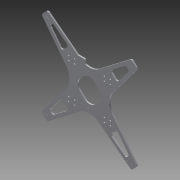
# Autodesk Inventor part: 6061 Bed holes no chamfer
Saved by Autodesk Inventor 2014 (Build 180170000, 170)
## iProperties
Created: 2016-05-10
Part Number: 6061 Bed holes no chamfer
Material: Aluminum 6061
Document SubType Name: Modeling
Designer: 101767
Density: 2.71 g/cm^3
Appearance: Aluminum - Flat
Mass: 1110.57 g
Surface Area: 1537.27 cm^2
Volume: 409.805 cm^3
Author: 101767
Autodesk Inventor part; units mm, degrees
ref_plane "YZ Plane" through (0, 0, 0) normal (1, 0, 0) x (0, 1, 0)
ref_plane "XZ Plane" through (0, 0, 0) normal (0, 1, 0) x (-1, 0, 0)
ref_plane "XY Plane" through (0, 0, 0) normal (0, 0, 1) x (1, 0, 0)
sketch "Plate" plane through (0, 0, 0) normal (0, 0, 1) x (1, 0, 0)
  line L0 (-200, -200) -> (200, -200) construction
  line L1 (200, -200) -> (200, 200) construction
  line L2 (200, 200) -> (-200, 200) construction
  line L3 (-200, 200) -> (-200, -200) construction
  line L4 (-200, -200) -> (200, 200) construction
  line L5 (200, -200) -> (-200, 200) construction
  line L6 (0, 0) -> (0, 420.657) construction
  line L7 (0, 0) -> (461.6465, 0) construction
  line L8 (0, 202) -> (202, 202) construction
  line L9 (202, 202) -> (202, 0) construction
  line L10 (74.8189, 0) -> (251.7605, 230.5948) construction
  line L11 (254.8388, 145.1612) -> (158.001, 241.999) construction
  line L12 (252.9755, 175.3088) -> (179.3809, 248.9034) construction
  line L13 (74.8189, 0) -> (228.2843, 200)
  line L14 (200, 200) -> (231.4665, 231.4665) construction
  line L15 (228.2843, 200) -> (214.1421, 214.1421)
  line L16 (200, 228.2843) -> (214.1421, 214.1421)
  line L17 (200, 228.2843) -> (0, 74.8189)
  line L18 (-74.8189, 0) -> (-228.2843, 200)
  line L19 (-228.2843, 200) -> (-214.1421, 214.1421)
  line L20 (-200, 228.2843) -> (-214.1421, 214.1421)
  line L21 (-200, 228.2843) -> (0, 74.8189)
  line L22 (74.8189, 0) -> (228.2843, -200)
  line L23 (228.2843, -200) -> (214.1421, -214.1421)
  line L24 (200, -228.2843) -> (214.1421, -214.1421)
  line L25 (200, -228.2843) -> (0, -74.8189)
  line L26 (-200, -228.2843) -> (0, -74.8189)
  line L27 (-200, -228.2843) -> (-214.1421, -214.1421)
  line L28 (-228.2843, -200) -> (-214.1421, -214.1421)
  line L29 (-74.8189, 0) -> (-228.2843, -200)
  dimension "d63" = 0
  dimension "d133" = 15
  dimension "d12" = 200
  dimension "d79" = 200
  dimension "d80" = 2
  dimension "d81" = 2
  dimension "d83" = 20
  dimension "d84" = 7.5
  dimension "d85" = 20
  dimension "d86" = 7.5
  constraints: 60 end point, 12 symmetric about line, 9 point on line, 5 parallel, 5 perpendicular, 2 midpoint, 1 horizontal
  measures "d12" distance between parallel lines of L7 L2
  measures "d79" distance from line of L1.end L6
  measures "d80" distance between parallel lines of L2 L8
  measures "d81" distance between parallel lines of L1 L9
  measures "d83" distance between parallel lines of L11 L12
  measures "d84" angle of L10 L4
  measures "d85" distance from line of L14 L13.end
  measures "d86" angle of L4 L17
extrude "Base" add sketch "Plate" along normal blind 6.35
sketch "Sketch3" plane through (0, 0, 0) normal (0, 0, 1) x (1, 0, 0)
  line L0 (-70.7107, 0) -> (0, 70.7107)
  line L1 (0, 70.7107) -> (70.7107, 0)
  line L2 (70.7107, 0) -> (0, -70.7107)
  line L3 (0, -70.7107) -> (-70.7107, 0)
  line L4 (-70.7107, 0) -> (70.7107, 0) construction
  line L5 (0, 70.7107) -> (0, -70.7107) construction
  point P0 (0, 0)
  dimension "d76" = 90
  dimension "d77" = 100
  constraints: 12 end point, 2 midpoint, 2 parallel, 1 perpendicular, 1 vertical
  measures "d76" angle of L4 L5
  measures "d77" distance of L0.end L1.end
extrude "Center hole" cut sketch "Sketch3" along normal through all
fillet "Fillet2" radius 75 4 edges at (0, 74.8189, 3.175) (-74.8189, 0, 3.175) (0, -74.8189, 3.175) (74.8189, 0, 3.175)
fillet "Fillet3" radius 35 4 edges at (-70.7107, 0, 3.175) (0, 70.7107, 3.175) (70.7107, 0, 3.175) (0, -70.7107, 3.175)
sketch "Sketch7" plane through (0, 0, 0) normal (0, 0, 1) x (1, 0, 0)
  line L0 (-255.2647, 85) -> (41.6783, 85) construction
  line L1 (-85, 158.0112) -> (-85, -43.0353) construction
  line L2 (-97.5, 95.5) -> (-100.5, 95.5) construction
  line L3 (-97.5, 98.125) -> (-100.5, 98.125)
  line L4 (-100.5, 92.875) -> (-97.5, 92.875)
  arc A0 (-97.5, 92.875) -> (-97.5, 98.125) centre (-97.5, 95.5) ccw
  arc A1 (-100.5, 98.125) -> (-100.5, 92.875) centre (-100.5, 95.5) ccw
  line L5 (-69.5, 98.125) -> (-72.5, 98.125)
  line L6 (-72.5, 92.875) -> (-69.5, 92.875)
  arc A2 (-69.5, 92.875) -> (-69.5, 98.125) centre (-69.5, 95.5) ccw
  arc A3 (-72.5, 98.125) -> (-72.5, 92.875) centre (-72.5, 95.5) ccw
  line L7 (-97.5, 77.125) -> (-100.5, 77.125)
  line L8 (-100.5, 71.875) -> (-97.5, 71.875)
  arc A4 (-97.5, 71.875) -> (-97.5, 77.125) centre (-97.5, 74.5) ccw
  arc A5 (-100.5, 77.125) -> (-100.5, 71.875) centre (-100.5, 74.5) ccw
  line L9 (-69.5, 77.125) -> (-72.5, 77.125)
  line L10 (-72.5, 71.875) -> (-69.5, 71.875)
  arc A6 (-69.5, 71.875) -> (-69.5, 77.125) centre (-69.5, 74.5) ccw
  arc A7 (-72.5, 77.125) -> (-72.5, 71.875) centre (-72.5, 74.5) ccw
  point P0 (0, 0)
  point P1 (-99, 95.5)
  dimension "d48" = 85
  dimension "d49" = 85
  dimension "d51" = 10.5
  dimension "d52" = 2.625
  dimension "d53" = 3
  dimension "d54" = 14
  dimension "d57" = 28
  dimension "d60" = 21
  constraints: 24 end point, 16 point on circle, 8 centre point, 4 tangent, 2 horizontal, 2 parallel, 1 midpoint, 1 perpendicular, 1 vertical, 30 other
  measures "d48" distance from line of L1 point (0, 0)
  measures "d49" distance from line of point (0, 0) L0
  measures "d51" distance from line of L0 point (-99, 95.5)
  measures "d52" radius of A1
  measures "d53" distance of L2.start L2.end
  measures "d54" distance from line of L1 point (-99, 95.5)
  measures "d57" distance of L3.start L5.start
  measures "d60" distance of L3.start L7.start
extrude "M5 Bearing Holes" cut sketch "Sketch7" along normal through all both and the other way through all
pattern_linear "Rectangular Pattern1" count 2 spacing 170 along (1, 0, 0) count 2 spacing 170 along (0, -1, 0) of "M5 Bearing Holes"
fillet "Fillet4" radius 10 8 edges at (200, 228.2843, 3.175) (228.2843, 200, 3.175) (228.2843, -200, 3.175) (200, -228.2843, 3.175) (-200, -228.2843, 3.175) (-228.2843, -200, 3.175) (-200, 228.2843, 3.175) (-228.2843, 200, 3.175)
sketch "Sketch11" plane through (0, 0, 0) normal (0, 0, 1) x (1, 0, 0)
  circle A0 centre (179.8878, 202) radius 1.65 projected
  circle A1 centre (202, 179.8878) radius 1.65 projected
  point P0 (0, 0)
  constraints: 2 coincident
hole "M3 holes" at (179.8878, 202, 0) at (202, 179.8878, 0) direction (0, 0, 1) diameter 2.5 end through all
sketch "Sketch12" plane through (0, 0, 0) normal (0, 0, 1) x (1, 0, 0)
  arc A0 (202, 199.8) -> (199.8, 202) centre (202, 202) ccw projected
  point P0 (0, 0)
  constraints: 1 coincident
hole "M4 hole" at (202, 202, 0) direction (0, 0, 1) diameter 3.3 end through all
pattern_circular "Circular Pattern1" count 4 over 360 about axis through (0, 0, -10) along (0, 0, 1) of "M3 holes", "M4 hole"
sketch "Sketch14" plane through (0, 0, 0) normal (0, 0, 1) x (1, 0, 0)
  line L0 (0, 0) -> (-162.672, 0) construction
  point P0 (-7, 75)
  point P1 (-7, -75)
  dimension "d117" = 7
  dimension "d118" = 75
  constraints: 2 end point, 1 horizontal, 1 symmetric about line
  measures "d117" horizontal distance of L0.start point (-7, 75)
  measures "d118" vertical distance of L0.start point (-7, 75)
hole "Hole5" at (-7, 75, 0) at (-7, -75, 0) direction (0, 0, 1) diameter 4.2 end through all
sketch "Sketch17" plane through (0, 0, 0) normal (0, 0, 1) x (1, 0, 0)
  line L0 (-200, -200) -> (200, 200) construction
  line L1 (254.8388, 145.1612) -> (158.001, 241.999) construction
  line L2 (182.3223, 182.3223) -> (174.6892, 189.9555)
  line L3 (174.6892, 189.9555) -> (98.6702, 131.6241)
  line L4 (98.6702, 131.6241) -> (115.1472, 115.1472)
  line L5 (193.0425, 222.9456) -> (45.6571, 109.8528) construction
  line L6 (182.3223, 182.3223) -> (189.9555, 174.6892)
  line L7 (189.9555, 174.6892) -> (131.6241, 98.6702)
  line L8 (131.6241, 98.6702) -> (115.1472, 115.1472)
  point P0 (0, 0)
  dimension "d133" = 15
  dimension "d134" = 25
  dimension "d135" = 95
  constraints: 12 end point, 2 parallel, 2 point on line, 2 symmetric about line, 1 perpendicular
  measures "d133" distance between parallel lines of L5 L3
  measures "d134" distance between parallel lines of L2 L1
  measures "d135" distance between parallel lines of L2 L4
extrude "Extrusion4" cut sketch "Sketch17" along normal through all
fillet "Fillet5" radius 10 4 edges at (174.6892, 189.9555, 3.175) (189.9555, 174.6892, 3.175) (131.6241, 98.6702, 3.175) (98.6702, 131.6241, 3.175)
pattern_circular "Circular Pattern2" count 4 over 360 about axis through (0, 0, -10) along (0, 0, 1) of "Extrusion4", "Fillet5"
sketch "Sketch18" plane through (0, 0, 0) normal (0, 0, 1) x (1, 0, 0)
  arc A0 (-45.6571, 109.8528) -> (45.6571, 109.8528) centre (0, 169.3543) ccw construction
  line L0 (-20, 97.0701) -> (-20, 117.5)
  line L1 (-20, 117.5) -> (-55.6231, 117.5)
  line L2 (-69.5, 100.125) -> (-72.5, 100.125) projected
  arc A1 (-69.5, 92.875) -> (-69.5, 98.125) centre (-69.5, 95.5) ccw construction
  line L3 (-45.6571, 109.8528) -> (-193.0425, 222.9456) construction
  line L4 (-55.6231, 117.5) -> (-45.6571, 109.8528)
  arc A2 (-45.6571, 109.8528) -> (-20, 97.0701) centre (0, 169.3543) ccw
  point P0 (0, 0)
  dimension "d144" = 20
  dimension "d146" = 22
  constraints: 6 end point, 3 point on circle, 1 centre point, 1 collinear, 1 concentric, 1 parallel, 1 perpendicular, 1 point on line, 1 tangent, 1 vertical
  measures "d144" distance from line of L0 point (0, 0)
  measures "d146" distance from line of L1 A1.centre
extrude "Limit nub" add sketch "Sketch18" along normal up to surface (6.35 mm away)
fillet "Fillet6" radius 5 3 edges at (-55.6231, 117.5, 3.175) (-20, 97.0701, 3.175) (-20, 117.5, 3.175)
body "Solid1"
